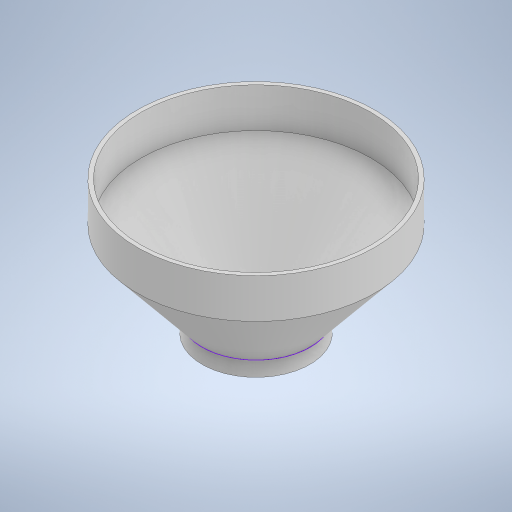
# Autodesk Inventor part: Widefield_LightShieldCone
Saved by Autodesk Inventor 2023 (Build 270158000, 158)
## iProperties
Created: 2023-02-09
Part Number: Widefield_LightShieldCone
Material: Generic
Document SubType Name: Modeling
Designer: User
Density: 1 g/cm^3
Appearance: Default
Author: User
Autodesk Inventor part; units mm, degrees
ref_plane "YZ Plane" through (0, 0, 0) normal (1, 0, 0) x (0, 1, 0)
ref_plane "XZ Plane" through (0, 0, 0) normal (0, 1, 0) x (-1, 0, 0)
ref_plane "XY Plane" through (0, 0, 0) normal (0, 0, 1) x (1, 0, 0)
sketch "Sketch1" plane through (0, 0, 0) normal (0, 1, 0) x (-1, 0, 0)
  circle A0 centre (0, 0) radius 6.3
  circle A1 centre (0, 0) radius 6.8
  dimension "d0" = 12.6
  dimension "d1" = 13.6
  constraints: 2 centre point, 2 coincident
  measures "d0" diameter of A0
  measures "d1" diameter of A1
extrude "Extrusion1" add sketch "Sketch1" along normal blind 1.9
sketch "Sketch2" plane through (0, 1.9, 0) normal (0, 1, 0) x (1, 0, 0)
  circle A0 centre (0, 0) radius 6.8
  constraints: 1 centre point
ref_plane "Work Plane1" through (0, 11.9, 0) normal (0, 1, 0) x (1, 0, 0)
sketch "Sketch3" plane through (0, 11.9, 0) normal (0, 1, 0) x (1, 0, 0)
  circle A0 centre (0, 0) radius 15
  dimension "d6" = 30
  constraints: 1 centre point, 1 coincident
  measures "d6" diameter of A0
loft "Loft1" add profiles "Sketch3" section 1 edges at (6.8, 1.9, 0)
sketch "Sketch4" plane through (0, 1.9, 0) normal (0, -1, 0) x (1, 0, 0)
  circle A0 centre (0, 0) radius 5.75
  dimension "d12" = 11.5
  constraints: 1 centre point, 1 coincident
  measures "d12" diameter of A0
sketch "Sketch5" plane through (0, 11.9, 0) normal (0, 1, 0) x (1, 0, 0)
  circle A0 centre (0, 0) radius 14.5
  dimension "d13" = 29
  constraints: 1 centre point, 1 coincident
  measures "d13" diameter of A0
loft "Loft2" cut profiles "Sketch4", "Sketch5"
sketch "Sketch6" plane through (0, 11.9, 0) normal (0, 1, 0) x (1, 0, 0)
  circle A0 centre (0, 0) radius 14.5
  circle A1 centre (0, 0) radius 15
  constraints: 2 centre point, 2 coincident
extrude "Extrusion2" add sketch "Sketch6" along normal blind 5
body "Solid1"
